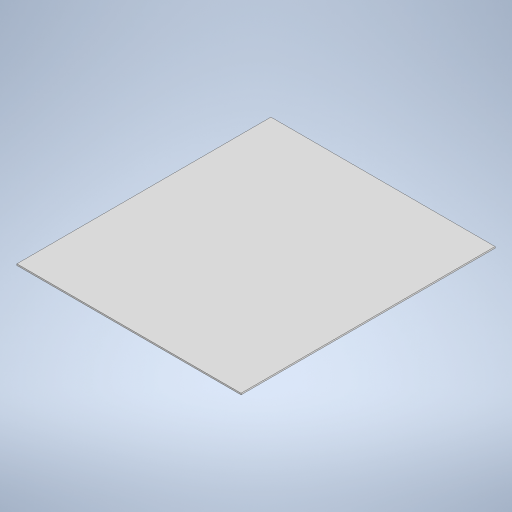
# Autodesk Inventor part: BungaCamp-Layout
Saved by Autodesk Inventor 2023 (Build 270158000, 158)
## iProperties
Created: 2024-07-15
Part Number: BungaCamp-Layout
Material: Generic
Document SubType Name: Modeling
Designer: incep
Density: 1 g/cm^3
Appearance: Default
Author: incep
Autodesk Inventor part; units mm, degrees
ref_plane "YZ Plane" through (0, 0, 0) normal (1, 0, 0) x (0, 1, 0)
ref_plane "XZ Plane" through (0, 0, 0) normal (0, 1, 0) x (-1, 0, 0)
ref_plane "XY Plane" through (0, 0, 0) normal (0, 0, 1) x (1, 0, 0)
sketch "Sketch1" plane through (0, 0, 0) normal (0, 1, 0) x (-1, 0, 0)
  line L0 (7500, -8500) -> (-7500, -8500)
  line L1 (-7500, -8500) -> (-7500, 8500)
  line L2 (-7500, 8500) -> (7500, 8500)
  line L3 (7500, 8500) -> (7500, -8500)
  line L4 (-2275.6359, -3661.1722) -> (162.7641, -3661.1722)
  line L5 (162.7641, -3661.1722) -> (1381.9641, -5772.8885)
  line L6 (1381.9641, -5772.8885) -> (162.7641, -7884.6049)
  line L7 (162.7641, -7884.6049) -> (-2275.6359, -7884.6049)
  line L8 (-2275.6359, -7884.6049) -> (-3494.8359, -5772.8885)
  line L9 (-3494.8359, -5772.8885) -> (-2275.6359, -3661.1722)
  line L10 (-5986.3012, -586.0191) -> (-3547.9012, -586.0191)
  line L11 (-3547.9012, -586.0191) -> (-2328.7012, -2697.7354)
  line L12 (-2328.7012, -2697.7354) -> (-3547.9012, -4809.4518)
  line L13 (-3547.9012, -4809.4518) -> (-5986.3012, -4809.4518)
  line L14 (-5986.3012, -4809.4518) -> (-7205.5012, -2697.7354)
  line L15 (-7205.5012, -2697.7354) -> (-5986.3012, -586.0191)
  line L16 (-404, 4452) -> (-6500, 4452)
  line L17 (-6500, 4452) -> (-6500, 7500)
  line L18 (-6500, 7500) -> (-404, 7500)
  line L19 (-404, 7500) -> (-404, 4452)
  line L20 (-404, 904) -> (-6500, 904)
  line L21 (-6500, 904) -> (-6500, 3952)
  line L22 (-6500, 3952) -> (-404, 3952)
  line L23 (-404, 3952) -> (-404, 904)
  line L24 (4225.0332, -7263.1726) -> (1725.0332, -7263.1726)
  line L25 (1725.0332, -7263.1726) -> (1725.0332, -263.1726)
  line L26 (1725.0332, -263.1726) -> (4225.0332, -263.1726)
  line L27 (4225.0332, -263.1726) -> (4225.0332, -7263.1726)
  line L28 (2839.1001, 1663.417) -> (339.1001, 1663.417)
  line L29 (339.1001, 1663.417) -> (339.1001, 5963.417)
  line L30 (339.1001, 5963.417) -> (2839.1001, 5963.417)
  line L31 (2839.1001, 5963.417) -> (2839.1001, 1663.417)
  line L32 (7267.7679, -7967.4048) -> (4767.7679, -7967.4048)
  line L33 (4767.7679, -7967.4048) -> (4767.7679, -3667.4048)
  line L34 (4767.7679, -3667.4048) -> (7267.7679, -3667.4048)
  line L35 (7267.7679, -3667.4048) -> (7267.7679, -7967.4048)
  line L36 (7267.7679, -2667.4048) -> (4767.7679, -2667.4048)
  line L37 (4767.7679, -2667.4048) -> (4767.7679, 1632.5952)
  line L38 (4767.7679, 1632.5952) -> (7267.7679, 1632.5952)
  line L39 (7267.7679, 1632.5952) -> (7267.7679, -2667.4048)
  line L40 (6469.8057, 6878.7001) -> (4469.8057, 6878.7001)
  line L41 (4469.8057, 6878.7001) -> (4469.8057, 2878.7001)
  line L42 (4469.8057, 2878.7001) -> (6469.8057, 2878.7001)
  line L43 (6469.8057, 2878.7001) -> (6469.8057, 6878.7001)
  line L44 (6249.8685, 4749.3609) -> (5634.674, 4749.3609) construction
  line L45 (5634.674, 4749.3609) -> (5634.674, 4905.6819) construction
  line L46 (5634.674, 4905.6819) -> (6249.8685, 4905.6819) construction
  line L47 (6249.8685, 4905.6819) -> (6249.8685, 4749.3609) construction
  line L48 (6251.456, 4750.9484) -> (5636.2615, 4750.9484) construction
  line L49 (5636.2615, 4750.9484) -> (5636.2615, 4907.2694) construction
  line L50 (5636.2615, 4907.2694) -> (6251.456, 4907.2694) construction
  line L51 (6251.456, 4907.2694) -> (6251.456, 4750.9484) construction
  line L52 (3797.5267, -3823.2725) -> (3797.5267, -4237.535) construction
  line L53 (3797.5267, -4237.535) -> (2323.9448, -4237.535) construction
  line L54 (2323.9448, -4237.535) -> (2323.9448, -3823.2725) construction
  line L55 (2323.9448, -3823.2725) -> (3797.5267, -3823.2725) construction
  line L56 (2391.2927, 4139.6846) -> (2391.2927, 3725.4221) construction
  line L57 (2391.2927, 3725.4221) -> (917.7109, 3725.4221) construction
  line L58 (917.7109, 3725.4221) -> (917.7109, 4139.6846) construction
  line L59 (917.7109, 4139.6846) -> (2391.2927, 4139.6846) construction
  line L60 (6794.0548, -134.534) -> (6794.0548, -4844.324) construction
  line L61 (6794.0548, -4844.324) -> (5320.473, -4844.324) construction
  line L62 (5320.473, -4844.324) -> (5320.473, -134.534) construction
  line L63 (5320.473, -134.534) -> (6794.0548, -134.534) construction
  line L64 (417.146, -5565.7573) -> (417.146, -5980.0198) construction
  line L65 (417.146, -5980.0198) -> (-1056.4359, -5980.0198) construction
  line L66 (-1056.4359, -5980.0198) -> (-1056.4359, -5565.7573) construction
  line L67 (-1056.4359, -5565.7573) -> (417.146, -5565.7573) construction
  line L68 (-3888.6954, -3064.2354) -> (-3888.6954, -3478.498) construction
  line L69 (-3888.6954, -3478.498) -> (-5362.2773, -3478.498) construction
  line L70 (-5362.2773, -3478.498) -> (-5362.2773, -3064.2354) construction
  line L71 (-5362.2773, -3064.2354) -> (-3888.6954, -3064.2354) construction
  line L72 (6746.7668, 382.2846) -> (6746.7668, -31.9779) construction
  line L73 (6746.7668, -31.9779) -> (5273.185, -31.9779) construction
  line L74 (5273.185, -31.9779) -> (5273.185, 382.2846) construction
  line L75 (5273.185, 382.2846) -> (6746.7668, 382.2846) construction
  line L76 (-2167.1387, 5835.591) -> (-2167.1387, 5421.3284) construction
  line L77 (-2167.1387, 5421.3284) -> (-3640.7205, 5421.3284) construction
  line L78 (-3640.7205, 5421.3284) -> (-3640.7205, 5835.591) construction
  line L79 (-3640.7205, 5835.591) -> (-2167.1387, 5835.591) construction
  line L80 (-2493.5133, 1971.221) -> (-2493.5133, 1556.9585) construction
  line L81 (-2493.5133, 1556.9585) -> (-3967.0952, 1556.9585) construction
  line L82 (-3967.0952, 1556.9585) -> (-3967.0952, 1971.221) construction
  line L83 (-3967.0952, 1971.221) -> (-2493.5133, 1971.221) construction
  point P0 (0, 0)
  point P1 (0, -8500)
  point P2 (-7500, 0)
  point P3 (-1056.4359, -5772.8885)
  point P4 (-4767.1012, -2697.7354)
  dimension "d0" = 15000
  dimension "d1" = 17000
  dimension "d2" = 2438.4
  dimension "d3" = 6096
  dimension "d4" = 3048
  dimension "d5" = 1000
  dimension "d6" = 500
  dimension "d7" = 2500
  dimension "d8" = 7000
  dimension "d10" = 2500
  dimension "d11" = 4300
  dimension "d14" = 1000
  dimension "d15" = 1000
  dimension "d16" = 4000
  dimension "d17" = 2000
  constraints: 88 end point, 16 parallel, 9 horizontal, 7 equal length, 7 perpendicular, 3 midpoint, 1 collinear, 1 horizontal alignment, 1 point on line, 1 vertical alignment, 45 other
  measures "d0" distance of L0.start L0.end
  measures "d1" distance of L2.end L0.start
  measures "d2" distance of L6.end L7.end
  measures "d3" distance of L17.end L18.end
  measures "d4" distance of L16.end L17.end
  measures "d5" distance between parallel lines of L18 L2
  measures "d6" distance between parallel lines of L22 L16
  measures "d7" distance of L24.start L24.end
  measures "d8" distance of L26.end L24.start
  measures "d10" distance of L28.start L28.end
  measures "d11" distance of L30.end L28.start
  measures "d14" distance between parallel lines of L34 L36
  measures "d15" distance between parallel lines of L1 L17
  measures "d16" distance of L40.end L41.end
  measures "d17" distance of L41.end L42.end
extrude "Extrusion1" add sketch "Sketch1" against normal blind 100 contours L0 L1 L2 L3 | L4 L5 L6 L7 L8 L9 | L10 L11 L12 L13 L14 L15 | L16 L17 L18 L19 | L20 L21 L22 L23 | L24 L25 L26 L27 | L28 L29 L30 L31 | L32 L33 L34 L35 | L36 L37 L38 L39 | L43 L42 L41 L40
body "Solid1"
